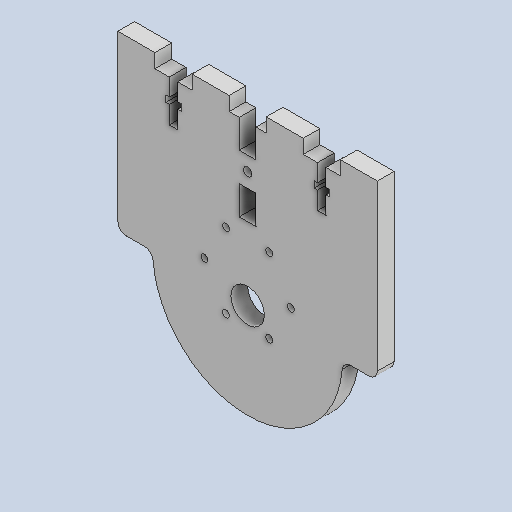
# Autodesk Inventor part: motor3
Saved by Autodesk Inventor 2023.1 (Build 271208000, 208)
## iProperties
Created: 2023-03-14
Part Number: motor3
Material: Типовые
Document SubType Name: Modeling
Designer: User
Density: 1 g/cm^3
Appearance: По умолчанию
Author: User
Autodesk Inventor part; units mm, degrees
ref_plane "YZ Plane" through (0, 0, 0) normal (1, 0, 0) x (0, 1, 0)
ref_plane "XZ Plane" through (0, 0, 0) normal (0, 1, 0) x (-1, 0, 0)
ref_plane "РабПлоскость1" through (89.2173, 100.7825, 86.5043) normal (0, 0, -1) x (-1, 0, 0)
sketch "Эскиз1" plane through (89.2173, 100.7825, 86.5043) normal (0, 0, -1) x (-1, 0, 0)
  line L0 (0, 7.6342) -> (-13.2857, 7.6342) construction
  line L1 (0, 7.6342) -> (0, 13.6342) projected
  line L2 (-13.2857, 13.6342) -> (0, 13.6342) projected
  line L3 (-13.2857, 7.6342) -> (-13.2857, 13.6342) projected
  line L4 (-26.5714, 7.6342) -> (-39.8571, 7.6342) construction
  line L5 (-26.5714, 7.6342) -> (-26.5714, 13.6342) projected
  line L6 (-39.8571, 13.6342) -> (-26.5714, 13.6342) projected
  line L7 (-39.8571, 7.6342) -> (-39.8571, 13.6342) projected
  line L8 (-53.1429, 7.6342) -> (-66.4286, 7.6342) construction
  line L9 (-53.1429, 7.6342) -> (-53.1429, 13.6342) projected
  line L10 (-66.4286, 13.6342) -> (-53.1429, 13.6342) projected
  line L11 (-66.4286, 7.6342) -> (-66.4286, 13.6342) projected
  line L12 (-79.7143, 7.6342) -> (-93, 7.6342) construction
  line L13 (-79.7143, 7.6342) -> (-79.7143, 13.6342) projected
  line L14 (-93, 13.6342) -> (-79.7143, 13.6342) projected
  line L15 (-93, 7.6342) -> (-93, 13.6342) projected
  line L16 (-13.2857, 7.6342) -> (-26.5714, 7.6342)
  line L17 (-39.8571, 7.6342) -> (-53.1429, 7.6342)
  line L18 (-66.4286, 7.6342) -> (-79.7143, 7.6342)
  line L19 (0, 7.6342) -> (0, -46.3658)
  line L20 (-3, -49.3658) -> (-9.6218, -49.3658)
  line L21 (-93, 7.6342) -> (-93, -46.3658)
  line L22 (-90, -49.3658) -> (-83.3782, -49.3658)
  line L23 (-12.5, -49.3658) -> (-80.5, -49.3658) construction
  arc A0 (-80.3881, -52.1226) -> (-12.6119, -52.1226) centre (-46.5, -49.3658) ccw
  arc A1 (-9.6218, -49.3658) -> (-12.6119, -52.1226) centre (-9.6218, -52.3658) ccw
  arc A2 (-80.3881, -52.1226) -> (-83.3782, -49.3658) centre (-83.3782, -52.3658) ccw
  arc A3 (-93, -46.3658) -> (-90, -49.3658) centre (-90, -46.3658) ccw
  arc A4 (-3, -49.3658) -> (0, -46.3658) centre (-3, -46.3658) ccw
  circle A5 centre (-46.5, -49.2217) radius 6
  circle A6 centre (-62, -42.2217) radius 1.25
  circle A7 centre (-54.25, -55.6451) radius 1.25
  circle A8 centre (-38.75, -55.6451) radius 1.25
  circle A9 centre (-31, -42.2217) radius 1.25
  circle A10 centre (-38.75, -28.7983) radius 1.25
  circle A11 centre (-54.25, -28.7983) radius 1.25
  point P0 (89.2173, -100.7825)
  point P1 (-93, -49.3658)
  dimension "d0" = 57
  dimension "d1" = 34
  dimension "d2" = 3
  dimension "d3" = 6
  constraints: 16 end point, 12 centre point, 12 point on circle, 8 tangent, 4 point on line, 3 equal radius, 2 collinear, 2 equal length, 2 perpendicular, 2 vertical, 1 horizontal, 1 midpoint, 14 other
  measures "d0" distance of L12.end point (-93, -49.366)
  measures "d1" radius of A0
  measures "d2" radius of A1
  measures "d3" distance between parallel lines of L2 L0
ref_plane "РабПлоскость2" through (219.2173, 403.7825, -131.4957) normal (0, 0, -1) x (-1, 0, 0)
extrude "Выдавливание1" add sketch "Эскиз1" along normal blind 6
sketch "Эскиз2" plane through (89.2173, 100.7825, 86.5043) normal (0, 0, 1) x (1, 0, 0)
  circle A0 centre (46.5, -42.2217) radius 19
  line L0 (49.5, -2.555) -> (43.5, -2.555)
  line L1 (43.5, -2.555) -> (43.5, -12.8884) construction
  line L2 (43.5, -12.8884) -> (49.5, -12.8884)
  line L3 (49.5, -12.8884) -> (49.5, -2.555) construction
  line L4 (49.5, -12.8884) -> (46.5, -42.2217) construction
  line L5 (46.5, -42.2217) -> (43.5, -12.8884) construction
  line L6 (49.5, -12.8884) -> (43.5, -2.555) construction
  line L7 (43.5, -12.8884) -> (43.5, -23.2217)
  line L8 (43.5, -23.2217) -> (49.5, -23.2217)
  line L9 (49.5, -23.2217) -> (49.5, -12.8884)
  line L10 (43.5, -2.555) -> (43.5, 7.7783)
  line L11 (49.5, -2.555) -> (49.5, 7.7783)
  circle A1 centre (46.5, -7.7217) radius 1.5
  line L12 (18.4286, 7.7783) -> (18.4286, 13.7783) construction
  line L13 (21.4286, 7.7783) -> (21.4286, 13.7783) construction
  line L14 (71.5714, 7.7783) -> (71.5714, 13.7783) construction
  line L15 (74.5714, 7.7783) -> (74.5714, 13.7783) construction
  line L16 (43.5, 7.7783) -> (49.5, 7.7783)
  line L17 (18.4286, 7.7783) -> (18.4286, 1.4283)
  line L18 (18.4286, 1.4283) -> (17.1786, 1.4283)
  line L19 (17.1786, 1.4283) -> (17.1786, -0.8717)
  line L20 (17.1786, -0.8717) -> (18.4286, -0.8717)
  line L21 (18.4286, -0.8717) -> (18.4286, -7.2217)
  line L22 (18.4286, -7.2217) -> (21.4286, -7.2217)
  line L23 (21.4286, -7.2217) -> (21.4286, -0.8717)
  line L24 (21.4286, -0.8717) -> (22.6786, -0.8717)
  line L25 (22.6786, -0.8717) -> (22.6786, 1.4283)
  line L26 (22.6786, 1.4283) -> (21.4286, 1.4283)
  line L27 (21.4286, 1.4283) -> (21.4286, 7.7783)
  line L28 (18.4286, 7.7783) -> (21.4286, 7.7783)
  line L29 (46.5, 7.7783) -> (46.5, -2.555) construction
  line L30 (74.5714, 7.7783) -> (74.5714, 1.4283)
  line L31 (74.5714, 1.4283) -> (75.8214, 1.4283)
  line L32 (75.8214, 1.4283) -> (75.8214, -0.8717)
  line L33 (75.8214, -0.8717) -> (74.5714, -0.8717)
  line L34 (74.5714, -0.8717) -> (74.5714, -7.2217)
  line L35 (74.5714, -7.2217) -> (71.5714, -7.2217)
  line L36 (71.5714, -7.2217) -> (71.5714, -0.8717)
  line L37 (71.5714, -0.8717) -> (70.3214, -0.8717)
  line L38 (70.3214, -0.8717) -> (70.3214, 1.4283)
  line L39 (70.3214, 1.4283) -> (71.5714, 1.4283)
  line L40 (71.5714, 1.4283) -> (71.5714, 7.7783)
  line L41 (71.5714, 7.7783) -> (74.5714, 7.7783)
  line L42 (335, 7.7783) -> (-15, 7.7783) construction
  point P0 (-89.2173, -100.7825)
  dimension "d19" = 6
  dimension "d21" = 3
  dimension "d22" = 5.5
  dimension "d23" = 2.3
  dimension "d26" = 15
  constraints: 84 end point, 14 point on line, 10 perpendicular, 10 symmetric about line, 8 vertical, 5 equal length, 2 centre point, 2 horizontal, 2 midpoint, 2 parallel, 1 tangent, 16 other
  measures "d19" distance of L0.start L0.end
  measures "d21" diameter of A1
  measures "d22" distance between parallel lines of L19 L25
  measures "d23" distance between parallel lines of L24 L26
extrude "Выдавливание2" cut sketch "Эскиз2" against normal blind 6 contours L8 L7 L2 L9 | L0 L10 L16 L11 | A1 | L28 L27 L26 L25 L24 L23 L22 L21 L20 L19 L18 L17 | L30 L31 L32 L33 L34 L35 L36 L37 L38 L39 L40 L41
sketch "Эскиз4" plane through (168.9316, 114.4167, 86.5043) normal (0, 1, 0) x (1, 0, 0)
  line L0 (13.2857, 6) -> (10.2857, 6) projected
  line L1 (-79.7143, 0) -> (-79.7143, 6) projected
  line L2 (13.2857, 6) -> (-79.7143, 6)
  line L3 (-79.7143, 6) -> (-79.7143, 0)
  line L4 (-79.7143, 0) -> (13.2857, 0)
  line L5 (13.2857, 0) -> (13.2857, 6)
  point P0 (-168.9316, 86.5043)
  point P1 (10.2857, 6)
  point P2 (-79.7143, 6)
  constraints: 8 end point, 2 parallel, 1 horizontal, 1 perpendicular
extrude "Выдавливание3" cut sketch "Эскиз4" against normal blind 1
equation "\"d5\" = d3"
equation "\"d19\" = d3"
equation "\"d14\" = d3"
